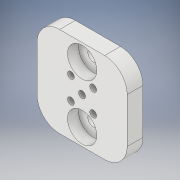
# Autodesk Inventor part: AA047
Saved by Autodesk Inventor 2017 SP1 (Build 210196100, 196)
## iProperties
Created: 2018-01-29
Part Number: AA047
Material: ABS Plastic
Document SubType Name: Modeling
Designer: Zach
Density: 1.06 g/cm^3
Appearance: CR White
Author: Zach
Autodesk Inventor part; units mm, degrees
ref_plane "YZ Plane" through (0, 0, 0) normal (1, 0, 0) x (0, 1, 0)
ref_plane "XZ Plane" through (0, 0, 0) normal (0, 1, 0) x (-1, 0, 0)
ref_plane "XY Plane" through (0, 0, 0) normal (0, 0, 1) x (1, 0, 0)
sketch "Sketch1" plane through (0, 0, 0) normal (0, 0, 1) x (1, 0, 0)
  line L0 (0, 0) -> (40, 0)
  line L1 (40, 0) -> (40, 40)
  line L2 (40, 40) -> (0, 40)
  line L3 (0, 40) -> (0, 0)
  line L4 (20, 32.5) -> (20, 7.5) construction
  circle A0 centre (20, 32.5) radius 2.5
  circle A1 centre (20, 7.5) radius 2.5
  point P0 (20, 20)
  point P1 (40, 20)
  point P2 (20, 40)
  dimension "d0" = 40
  dimension "d1" = 40
  dimension "d2" = 25
  dimension "d3" = 5
  dimension "d4" = 5
  constraints: 10 end point, 3 midpoint, 2 centre point, 2 coincident, 2 parallel, 1 horizontal, 1 horizontal alignment, 1 perpendicular, 1 vertical, 1 vertical alignment
  measures "d0" distance of L2.end L1.end
  measures "d1" distance of L1.end L0.end
  measures "d2" distance of L4.start L4.end
  measures "d3" diameter of A0
  measures "d4" diameter of A1
extrude "Extrusion1" add sketch "Sketch1" along normal blind 7
sketch "Sketch2" plane through (0, 0, 7) normal (0, 0, 1) x (1, 0, 0)
  circle A0 centre (20, 32.5) radius 2.5 projected
  circle A1 centre (20, 7.5) radius 2.5 projected
  circle A2 centre (20, 32.5) radius 6.5
  circle A3 centre (20, 7.5) radius 6.5
  point P0 (0, 0)
  dimension "d7" = 13
  dimension "d8" = 13
  constraints: 2 centre point, 2 coincident
  measures "d7" diameter of A2
  measures "d8" diameter of A3
extrude "Extrusion2" cut sketch "Sketch2" against normal blind 5
sketch "Sketch3" plane through (0, 0, 7) normal (0, 0, 1) x (1, 0, 0)
  circle A0 centre (20, 20) radius 1.5
  line L0 (40, 40) -> (0, 40) projected
  line L1 (40, 0) -> (40, 40) projected
  circle A1 centre (24.9497, 24.9497) radius 1.5
  line L2 (20, 20) -> (24.9497, 24.9497) construction
  line L3 (20, 20) -> (27, 20) construction
  circle A2 centre (15.0503, 24.9497) radius 1.5
  circle A3 centre (15.0503, 15.0503) radius 1.5
  circle A4 centre (24.9497, 15.0503) radius 1.5
  point P0 (0, 0)
  point P1 (20, 40)
  point P2 (40, 20)
  dimension "d11" = 3
  dimension "d12" = 3
  dimension "d13" = 45
  dimension "d14" = 7
  dimension "d17" = 360
  constraints: 5 centre point, 4 end point, 2 midpoint, 1 coincident, 1 equal length, 1 horizontal, 1 horizontal alignment, 1 vertical alignment, 9 other
  measures "d11" diameter of A0
  measures "d12" diameter of A1
  measures "d13" angle of L3 L2
  measures "d14" distance of L2.start L2.end
extrude "Extrusion3" cut sketch "Sketch3" against normal through all
fillet "Fillet1" radius 10 4 edges at (40, 40, 3.5) (40, 0, 3.5) (0, 40, 3.5) (0, 0, 3.5)
body "Solid1"
